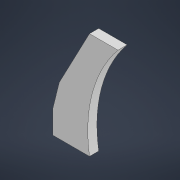
# Autodesk Inventor part: Base_Aerofoil
Saved by Autodesk Inventor 2022 (Build 260153000, 153)
## iProperties
Created: 2022-06-10
Part Number: Base_Aerofoil
Material: Generic
Document SubType Name: Modeling
Designer: Gugarauj07
Density: 1 g/cm^3
Appearance: Default
Author: Gugarauj07
Autodesk Inventor part; units mm, degrees
ref_plane "YZ Plane" through (0, 0, 0) normal (1, 0, 0) x (0, 1, 0)
ref_plane "XZ Plane" through (0, 0, 0) normal (0, 1, 0) x (-1, 0, 0)
ref_plane "XY Plane" through (0, 0, 0) normal (0, 0, 1) x (1, 0, 0)
sketch "Sketch1" plane through (0, 0, 0) normal (0, 0, 1) x (1, 0, 0)
  line L0 (0, 0) -> (80, 0)
  line L1 (0, 80) -> (0, 0)
  line L2 (40, 0) -> (160, 0) construction
  line L3 (0, 80) -> (80, 231.8222)
  line L4 (80, 231.8222) -> (142.1166, 231.8222)
  arc A0 (142.1166, 231.8222) -> (80, 0) centre (367.4632, 47.2076) ccw
  dimension "d2" = 240
  dimension "d4" = 80
  constraints: 10 end point, 3 horizontal, 2 point on circle, 1 centre point
  measures "d2" distance of L0.end L4.end
  measures "d4" distance of point (0, 0) L0.end
extrude "Extrusion1" add sketch "Sketch1" along normal blind 20
chamfer "Chamfer1" distance 30 angle 45 1 edges at (0, 80, 10)
body "Solid1"
